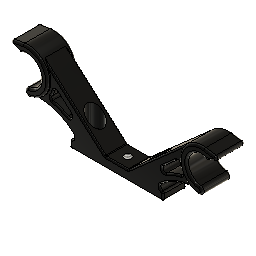
20021-018_payload-deck-clip (Autodesk Fusion 360 design; units mm, degrees)
Autodesk Fusion 360 part; units mm, degrees
sketch "Sketch1" plane through (0, 0, 0) normal (0, 1, 0) x (1, 0, 0)
  line L0 (0, 0) -> (0, -3.48)
  line L1 (0, -3.48) -> (-3.95, -3.48)
  line L2 (-3.95, -3.48) -> (-25.0839, -22.0844)
  arc A0 (-31.1242, -23.8546) -> (-29.1029, -9.1143) centre (-30, -16.5) ccw
  arc A1 (-32.0622, -20.8787) -> (-29.4164, -11.6953) centre (-30, -16.5) ccw
  arc A2 (-29.1029, -9.1143) -> (-29.4164, -11.6953) centre (-29.2597, -10.4048) ccw
  arc A3 (-29.1029, -9.1143) -> (-15.1821, -4.8007) centre (-26.9547, 8.5725) ccw
  arc A4 (-15.1821, -4.8007) -> (-15.975, -2.7) centre (-15.975, -3.9) ccw
  line L3 (-15.975, 0) -> (0, 0)
  line L4 (-31.1242, -23.8546) -> (-37.5, -22.88)
  line L5 (-37.5, -22.88) -> (-32.0622, -20.8787)
  line L6 (-15.975, 0) -> (-15.975, -2.7)
  line L7 (-15.1821, -4.8007) -> (-9.7287, 0) construction
  arc A5 (-23.1874, -11.1375) -> (-16.9838, -8.8418) centre (-26.9547, 8.5725) ccw
  arc A6 (-21.4123, -15.3084) -> (-23.1874, -11.1375) centre (-30, -16.5) ccw
  arc A7 (-15.8566, -10.4177) -> (-16.9838, -8.8418) centre (-16.5, -9.6868) ccw
  line L8 (-15.8566, -10.4177) -> (-21.4123, -15.3084)
  dimension "d1" = 3.48
  dimension "d2" = 3.95
  dimension "d3" = 15.975
  dimension "d4" = 1.2
  dimension "d5" = 4.84
  dimension "d7" = 2.6
  dimension "d9" = 30
  dimension "d10" = 16.5
  dimension "d11" = 2.7
  dimension "d12" = 2.8
  dimension "d14" = 37.5
  dimension "d21" = 22.88
  dimension "d35" = 2.25
  dimension "d36" = 2.66
  dimension "d37" = 3.83
  dimension "d38" = 16.5
  constraint coincident L0.start L3.end
  constraint vertical L0
  constraint perpendicular L0 L1
  constraint coincident L2.end A0
  constraint horizontal L3
  constraint tangent A3 A4
  constraint tangent A2 A3
  constraint tangent A0 A3
  constraint concentric A0 A1
  constraint tangent A1 A2
  constraint tangent A0 L4
  constraint perpendicular L3 L6
  constraint coincident A4.end L6.end
  constraint coincident A4.centre L6
  constraint coincident L3 L7.end
  constraint tangent A4 L7
  constraint parallel L2 L7
  constraint tangent L2 A0
  constraint coincident A3.centre A5.centre
  constraint coincident A0.centre A1.centre
  constraint tangent A7 L8
  constraint parallel L2 L8
  constraint tangent A5 A7
  measures "d1" distance of L0.start L0.end
  measures "d2" distance of L0.end L1.end
  measures "d3" distance of L0 L6
  measures "d4" radius of A4
  measures "d5" radius of A1
  measures "d7" distance of A0 A1
  measures "d9" distance of L0 A0.centre
  measures "d10" distance of A0.centre L3
  measures "d11" distance of L3.start A4.end
  measures "d12" distance of A1.start L4 L0.start
  measures "d14" distance of L0 L4.end
  measures "d21" distance of L3 L4.end
  measures "d35" distance of A3 A5
  measures "d36" distance of L2 L8 L0.start
  measures "d37" distance of A1 A6
  measures "d38" distance of L0 A7.centre
extrude "Extrude1" add sketch "Sketch1" along normal mid plane 7.94 contours L0 L1 L2 A0 A3 A4 L3 L6 makes body 1
extrude "Extrude2" add sketch "Sketch1" along normal mid plane 10 contours A0 A1 A2 L4 L5 bodies 1
fillet "Fillet2" radius 0.75 1 edges at (-37.5, 0, 22.88) on bodies 1
fillet "Fillet3" radius 0.7 15 edges at (-25.3492, -5, 17.84) (-30.5502, -5, 10.248) (-22.629, -5, 17.5107) (-32.8734, -5, 23.5872) (-35.2554, -5, 22.6537) (-33.4153, -5, 21.3766) (-33.4153, 5, 21.3766) (-35.2554, 5, 22.6537) (-32.8734, 5, 23.5872) (-22.629, 5, 17.5107) (-30.5502, 5, 10.248) (-25.3492, 5, 17.84) (-15.975, 0, 2.7) (-23.1874, 0, 11.1375) (-21.4123, 0, 15.3084) on bodies 1
fillet "Fillet4" radius 0.5 31 edges at (-3.95, 0, 3.48) (-1.975, 3.97, 3.48) (-1.975, -3.97, 3.48) (-14.517, -3.97, 12.7822) (-14.517, 3.97, 12.7822) (-7.9875, -3.97, 0) (-7.9875, 3.97, 0) (-15.975, 0, 0) (-15.975, 3.97, 1.0668) (-15.854, 3.97, 2.527) (-14.7928, 3.97, 3.6943) (-21.6813, 3.97, 8.446) (-21.6813, -3.97, 8.446) (-14.7928, -3.97, 3.6943) (-15.854, -3.97, 2.527) (-15.975, -3.97, 1.0668) (-32.0713, -4.8029, 21.1091) (-32.0622, 0, 20.8787) (-32.0713, 4.8029, 21.1091) (-19.5097, -3.97, 10.0621) (-22.6619, -3.97, 11.3319) (-22.0518, -3.97, 13.0367) (-21.1721, -3.97, 14.6599) (-18.1834, -3.97, 12.466) (-15.708, -3.97, 9.1203) (-22.0518, 3.97, 13.0367) (-21.1721, 3.97, 14.6599) (-18.1834, 3.97, 12.466) (-15.708, 3.97, 9.1203) (-19.5097, 3.97, 10.0621) (-22.6619, 3.97, 11.3319) on bodies 1
mirror "Mirror1" about plane through (0, 0, 0) normal (1, 0, 0) of bodies 1 makes body 2
combine "Combine1" operation add target body 1 tool bodies 2
ref_plane "WorkPlane1" through (0, 0, 6.7) normal (0, 0, 1) x (1, 0, 0)
sketch "Sketch2" plane through (0, 0, 6.7) normal (0, 0, 1) x (1, 0, 0)
  line L0 (15.475, 3.47) -> (-15.475, 3.47)
  line L1 (-15.475, 3.47) -> (-15.475, -3.47)
  line L2 (-15.475, -3.47) -> (15.475, -3.47)
  line L3 (15.475, -3.47) -> (15.475, 3.47)
  line L4 (-11.31, 0) -> (11.31, 0)
  dimension "d26" = 22.62
  constraint parallel L0 L4
  constraint midpoint origin L4
  measures "d26" distance of L4.start L4.end
hole "Hole1" at (-11.31, 0, 6.7) at (0, 0, 6.7) at (11.31, 0, 6.7) direction (0, 0, -1) diameter 2.529 end up to surface (6.7 mm away) counterbore diameter 5.5 counterbore depth 2.5 bodies 1
thread "Thread1" "ISO Metric profile 3.0 M3x0.5 6H"
extrude "Extrude3" cut 2 faces at (12.085, 1.3793, 6.7) (-10.535, 1.3793, 6.7) along direction (0, 0, 1) blind 24 on bodies 1 bodies 1
equation "d2 = ( 7.9 / 2 ) * 1 mm"
equation "d3 = ( 31.95 / 2 ) * 1 mm"
equation "d5 = ( 9.68 / 2 ) * 1 mm"
equation "d14 = ( 75 / 2 ) * 1 mm"
equation "d27 = 4.2 mm + 2.5 mm"
equation "d38 = ( 33 / 2 ) * 1 mm"
named bodies: "20021-018_payload-deck-clip"
